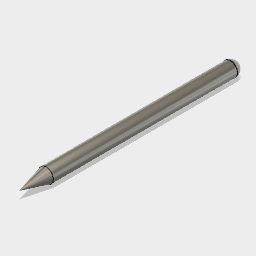
pen (Autodesk Fusion 360 design; units mm, degrees)
Autodesk Fusion 360 part; units mm, degrees
cylinder "圆柱体基本要素1" add diameter 8 height 100 placed x (0, 0, -1) y (0, 1, 0) z (1, 0, 0) at (0, 0, 0) makes body 1
sphere "球体基本要素1" add diameter 8 placed x (0, 0, -1) y (0, 1, 0) z (1, 0, 0) at (0, -4, 14) separate body makes body 2
move_body "对齐1" bodies 1 to x (0, 0, -1) y (0, 1, 0) z (1, 0, 0) at (0, -4, 114)
combine "合并1" operation add target body 1 tool bodies 2
sketch "草图3" plane through (0, 0, 0) normal (0, 0, 1) x (1, 0, 0)
  line L0 (-79, -58) -> (-75, -58)
  line L1 (-75, -58) -> (-75, -43)
  line L2 (-75, -43) -> (-79, -58)
revolve "旋转1" add sketch "草图3" angle 360 about axis through (-75, -58, 0) along (0, 1, 0) separate body makes body 3
move_body "对齐2" bodies 3 to x (1, 0, 0) y (0, 0, 1) z (0, -1, 0) at (75, -4, 172)
combine "合并2" operation add target body 1 tool bodies 3
